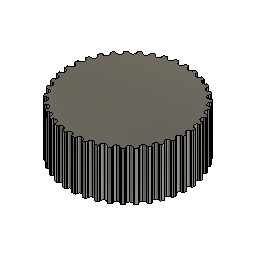
gear_39z (Autodesk Fusion 360 design; units mm, degrees)
Autodesk Fusion 360 part; units mm, degrees
sketch "Sketch1" plane through (0, 0, 0) normal (0, 0, 1) x (1, 0, 0) in component "gt2 pulley"
  circle A0 centre (0, 0) radius 12.4141 construction
  circle A1 centre (0, 0) radius 11.4101 construction
  line L0 (0, 0) -> (0, 12.4141) construction
  line L1 (0, 0) -> (0.9989, 12.3738) construction
  line L2 (0, 0) -> (1.4086, 12.3339) construction
  circle A2 centre (0, 0) radius 12.1601 construction
  arc A3 (0.3819, 12.0175) -> (0.4427, 11.7326) centre (1.3798, 12.0815) ccw
  circle A4 centre (0, 0) radius 12.0101 construction
  arc A5 (0.235, 12.1578) -> (0, 12.1601) centre (0, 0) ccw
  arc A6 (0.3819, 12.0175) -> (0.235, 12.1578) centre (0.2322, 12.0078) ccw
  arc A7 (0.4427, 11.7326) -> (0.9181, 11.3731) centre (0.9628, 11.9263) ccw
  arc A8 (0, 12.1601) -> (-0.235, 12.1578) centre (0, 0) ccw
  arc A9 (-0.235, 12.1578) -> (-0.3819, 12.0175) centre (-0.2322, 12.0078) ccw
  arc A10 (-0.4427, 11.7326) -> (-0.3819, 12.0175) centre (-1.3798, 12.0815) ccw
  arc A11 (-0.918, 11.3731) -> (-0.4427, 11.7326) centre (-0.9628, 11.9263) ccw
  arc A12 (0.9181, 11.3731) -> (-0.9181, 11.3731) centre (0, 0) ccw
  point P0 (1.3798, 12.0815)
  point P1 (0, 12.1601)
  dimension "d18" = 24.8282
  dimension "d19" = 4.615
  dimension "d22" = 1.004
  dimension "d24" = 0.75
  dimension "d26" = 1
  dimension "d27" = 0.15
  dimension "d28" = 0.15
  dimension "d47" = 0.555
  dimension "d52" = 3.812
  constraint coincident A0.centre A1.centre
  constraint coincident A0 L0.end
  constraint vertical L0
  constraint coincident A0 L1.end
  constraint coincident A0 L2.end
  constraint concentric A1 A2
  constraint coincident A1 A7.end
  constraint coincident L1 A7.end
  constraint coincident A2 P0
  constraint coincident L2 P0
  constraint coincident P0 A3.centre
  constraint coincident A2 P1
  constraint coincident L0 P1
  constraint concentric A2 A4
  constraint coincident P1 A5.end
  constraint coincident A4 A6.centre
  constraint coincident A3.start A6.start
  constraint tangent A3 A6
  constraint tangent A3 A7
  constraint symmetric L0 A7.end A12.end
  constraint symmetric L0 A3.start A9.end
  constraint symmetric L0 A3.end A10.start
  constraint symmetric L0 A3 A10
  constraint symmetric L0 A5.start A8.end
  constraint symmetric L0 P1 A5.end
  constraint symmetric L0 A5 A8
  constraint symmetric L0 A6 A9
  constraint symmetric L0 A7 A11
  constraint coincident A1 A11.start
  constraint tangent A1 A7
  constraint coincident L1 A7.centre
  measures "d18" diameter of A0
  measures "d19" angle of L0 L1
  measures "d22" distance of A0 A1
  measures "d24" distance of A1 A2
  measures "d26" radius of A3
  measures "d27" distance of A2 A4
  measures "d28" radius of A6
  measures "d47" radius of A7
extrude "Extrude1" add sketch "Sketch1" along normal blind 10 makes body 1
pattern_circular "C-Pattern1" count 39 over 360 about axis through (0, 0, 1.75) along (0, 0, 1) of bodies 1 makes body 2 at (-1.1215, 11.3548, 3.3333) makes body 3 at (-2.9285, 11.0279, 3.3333) makes body 4 at (-5.3927, 10.0553, 6.6667) makes body 5 at (-6.9358, 9.0601, 6.6667) makes body 6 at (-8.7076, 7.3734, 6.6667) makes body 7 at (-9.4479, 6.3974, 6.6667) makes body 8 at (-10.5944, 4.2365, 6.6667) makes body 9 at (-10.9875, 3.0764, 6.6667) makes body 10 at (-11.2186, 2.0819, 3.3333) makes body 11 at (-11.3963, -0.5614, 6.6667) makes body 12 at (-11.0147, -2.9777, 6.6667) makes body 13 at (-10.3944, -4.706, 6.6667) makes body 14 at (-9.83, -5.7932, 6.6667) makes body 15 at (-8.7734, -7.295, 6.6667) makes body 16 at (-7.0168, -8.9975, 6.6667) makes body 17 at (-6.0118, -9.6978, 6.6667) makes body 18 at (-5.1209, -10.1964, 3.3333) makes body 19 at (-3.4189, -10.8858, 3.3333) makes body 20 at (-1.6284, -11.2933, 3.3333) makes body 21 at (1.0198, -11.3644, 6.6667) makes body 22 at (2.0316, -11.2278, 3.3333) makes body 23 at (3.8063, -10.7565, 3.3333) makes body 24 at (6.1843, -9.5888, 6.6667) makes body 25 at (7.0167, -8.9976, 3.3333) makes body 26 at (8.9025, -7.1369, 6.6667) makes body 27 at (9.5048, -6.3126, 3.3333) makes body 28 at (10.7044, -3.9505, 6.6667) makes body 29 at (11.0147, -2.9778, 3.3333) makes body 30 at (11.3497, -1.1724, 3.3333) makes body 31 at (11.3141, 1.4766, 6.6667) makes body 32 at (11.1369, 2.482, 3.3333) makes body 33 at (10.5945, 4.2364, 3.3333) makes body 34 at (9.332, 6.5654, 6.6667) makes body 35 at (7.7181, 8.4037, 6.6667) makes body 36 at (6.2701, 9.5329, 6.6667) makes body 37 at (4.6597, 10.4152, 6.6667) makes body 38 at (4.2838, 10.5754, 3.3333) makes body 39 at (1.7295, 11.2782, 6.6667)
sketch "Sketch2" plane through (0, 0, 10) normal (0, 0, 1) x (-1, 0, 0)
  arc A0 (-7.5247, -9.3779) -> (-7.4916, -9.5783) centre (-7.3992, -9.4601) ccw
  arc A1 (-7.4916, -9.5783) -> (-7.1158, -9.8607) centre (0, 0) ccw
  arc A2 (-7.1158, -9.8607) -> (-6.9141, -9.8367) centre (-7.028, -9.7391) ccw
  arc A3 (-6.6944, -9.6455) -> (-6.9141, -9.8367) centre (-6.1548, -10.4874) ccw
  arc A4 (-6.0984, -9.6436) -> (-6.6944, -9.6455) centre (-6.3949, -10.1128) ccw
  arc A5 (-7.5663, -8.5406) -> (-6.0984, -9.6436) centre (0, 0) ccw
  arc A6 (-7.4022, -9.1137) -> (-7.5663, -8.5406) centre (-7.9343, -8.956) ccw
  arc A7 (-7.5247, -9.3779) -> (-7.4022, -9.1137) centre (-8.361, -8.8296) ccw
  circle A8 centre (0, 0) radius 11.4101
  constraint coincident A1.centre A5.centre
extrude "Extrude2" add sketch "Sketch2" against normal blind 10 contours A5 A8 bodies 1 2 3 4 5 6 7 8 9 10 11 12 13 14 15 16 17 18 19 20 21 22 23 24 25 26 27 28 29 30 31 32 33 34 35 36 37 38 39
extrude "Extrude4" [suppressed] in component "gt2 pulley"
pattern_circular "C-Pattern7" [suppressed] in component "gt2 pulley"
extrude "Extrude3" [suppressed] in component "gt2 pulley"
pattern_circular "C-Pattern6" [suppressed] in component "gt2 pulley"
extrude "Extrude2'" [suppressed] in component "gt2 pulley"
pattern_circular "C-Pattern5" [suppressed] in component "gt2 pulley"
extrude "Extrude1'" [suppressed] in component "gt2 pulley"
pattern_circular "C-Pattern4" [suppressed] in component "gt2 pulley"
pattern_circular "C-Pattern3" [suppressed] in component "gt2 pulley"
pattern_circular "C-Pattern2" [suppressed] in component "gt2 pulley"
pattern_circular "C-Pattern1'" [suppressed] in component "gt2 pulley"
copy_body "Body->Comp1" [suppressed] in component "Component"
copy_body "Body->Comp2" [suppressed] in component "Component'"
copy_body "Body->Comp3" [suppressed] in component "Component''"
copy_body "Body->Comp4" [suppressed] in component "Component'''"
copy_body "Body->Comp5" [suppressed] in component "Component''''"
copy_body "Body->Comp6" [suppressed] in component "Component'''''"
copy_body "Body->Comp7" [suppressed] in component "Component''''''"
copy_body "Body->Comp8" [suppressed] in component "Component'''''''"
copy_body "Body->Comp9" [suppressed] in component "Component''''''''"
copy_body "Body->Comp10" [suppressed] in component "Component'''''''''"
copy_body "Body->Comp11" [suppressed] in component "Component''''''''''"
copy_body "Body->Comp12" [suppressed] in component "Component'''''''''''"
copy_body "Body->Comp13" [suppressed] in component "Component''''''''''''"
copy_body "Body->Comp14" [suppressed] in component "Component'''''''''''''"
copy_body "Body->Comp15" [suppressed] in component "Component''''''''''''''"
copy_body "Body->Comp16" [suppressed] in component "Component'''''''''''''''"
copy_body "Body->Comp17" [suppressed] in component "Component''''''''''''''''"
copy_body "Body->Comp18" [suppressed] in component "Component'''''''''''''''''"
copy_body "Body->Comp19" [suppressed] in component "Component''''''''''''''''''"
copy_body "Body->Comp20" [suppressed] in component "Component'''''''''''''''''''"
component "gt2 pulley" placed x (1, 0, 0) y (0, 1, 0) z (0, 0, 1) at (0, 0, 0)
equation "NumTeeth = 39" comment "min 20"
equation "ToothPitch = 2 mm"
equation "PullyDia = NumTeeth * ToothPitch / PI"
equation "ToothAng = ( ( 360 / NumTeeth ) * 1 deg )"
equation "TransOffsetAngle = ToothAng * 0.2"
equation "Sholulder_Radius = 0.15 mm"
equation "Root_Radius = 0.555 mm"
equation "TransRadius = 1 mm"
equation "ToolHeight = 0.75 mm"
equation "PLD = 0.254 mm"
equation "d18 = PullyDia"
equation "d19 = ToothAng / 2"
equation "d22 = PLD + ToolHeight"
equation "d24 = ToolHeight"
equation "d26 = TransRadius"
equation "d27 = Sholulder_Radius"
equation "d31 = NumTeeth"
equation "d33 = NumTeeth"
equation "d35 = NumTeeth"
equation "d37 = NumTeeth"
equation "d41 = NumTeeth"
equation "d45 = NumTeeth"
equation "d47 = Root_Radius"
equation "d50 = NumTeeth"
